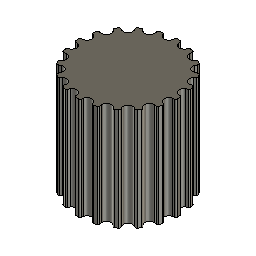
GT2-3M Generator (Autodesk Fusion 360 design; units mm, degrees)
Autodesk Fusion 360 part; units mm, degrees
sketch "Teeth" plane through (0, 0, 0) normal (0, 0, 1) x (1, 0, 0)
  circle A0 centre (0, 0) radius 9.5493
  arc A1 (0.5695, 8.5428) -> (1.2559, 7.9295) centre (1.3889, 8.769) ccw
  line L0 (0, 0) -> (0, 7.1835) construction
  line L1 (0, 0) -> (1.3889, 8.769) construction
  line L2 (0, 9.1683) -> (0, 9.5493)
  arc A2 (1.4938, 9.4317) -> (0, 9.5493) centre (0, 0) ccw
  arc A3 (0.2724, 9.1643) -> (0, 9.1683) centre (0, 0) ccw
  arc A4 (0.515, 8.919) -> (0.2724, 9.1643) centre (0.265, 8.9144) ccw
  arc A5 (0.515, 8.919) -> (0.5695, 8.5428) centre (2.0347, 8.9473) ccw
  line L3 (1.4938, 9.4317) -> (2.0963, 9.3363) construction
  line L4 (2.0347, 8.9473) -> (2.0963, 9.3363) construction
  arc A6 (1.2559, 7.9295) -> (2.0982, 8.3007) centre (1.3889, 8.769) ccw
  arc A7 (2.0982, 8.3007) -> (2.2664, 8.6416) centre (0.8297, 9.1381) ccw
  arc A8 (2.5728, 8.7999) -> (2.2664, 8.6416) centre (2.5026, 8.56) ccw
  arc A9 (2.8332, 8.7196) -> (2.5728, 8.7999) centre (0, 0) ccw
  line L5 (2.8332, 8.7196) -> (2.9509, 9.0819)
  arc A10 (2.9509, 9.0819) -> (1.4938, 9.4317) centre (0, 0) ccw
  dimension "d50" = 19.0986
  dimension "d59" = 9
  dimension "d67" = 0.381
  dimension "d68" = 0.25
  dimension "d69" = 1.521
  dimension "d71" = 0.61
  dimension "d72" = 0.85
  dimension "d73" = 1.52
  constraint coincident A0.centre L0.start
  constraint coincident A0 L2.end
  constraint parallel L0 L2
  constraint coincident A0 A2.start
  constraint collinear A1.centre A0.centre A2.start
  constraint coincident A1.centre L1.end
  constraint coincident L1 A1.end
  constraint vertical L0
  constraint coincident L0 L2.start
  constraint tangent A3 A4
  constraint tangent A4 A5
  constraint tangent A1 A5
  constraint tangent A0 L3
  constraint coincident A5.centre L4.start
  constraint coincident L3 L4.end
  constraint perpendicular L3 L4
  constraint coincident L3.end L4.end
  constraint symmetric A1 L1 A6
  constraint symmetric L1 L2.end L5.end
  constraint symmetric L1 A2.start L3.start
  constraint symmetric L1 A2 A10
  constraint symmetric L1 A1.end A6.start
  constraint symmetric L1 L2.start A9.start
  constraint symmetric L1 A3.start A8.start
  constraint symmetric L1 A3 A9
  constraint symmetric L1 A4.start A7.end
  constraint symmetric L1 A4 A8
  constraint symmetric L1 A1.start A6.end
  constraint symmetric L1 A5 A7
  measures "d50" diameter of A0
  measures "d59" angle of L0 L1
  measures "d67" distance of L2.end L2.start
  measures "d68" radius of A4
  measures "d69" distance of A2.start A1.end
  measures "d71" distance of A2.start L3.end
  measures "d72" radius of A1
  measures "d73" radius of A5
extrude "Extrude1" add sketch "Teeth" along normal mid plane 18.5
extrude "Extrude3" cut sketch "Teeth" along normal through all and the other way through all contours A0 A1 L2 A2 A3 A4 A5 A6 A7 A8 A9 L5 A10
pattern_circular "C-Pattern1" count 20 over 360 about axis through (0, 0, 0) along (0, 0, 1) of "Extrude3"
equation "p = 3 mm"
equation "Dr = 0.2 in" comment "0.13 for #25, 0.2 for #35"
equation "Ds = 1.0005 * Dr + 0.003 in"
equation "n = 20" comment "Number of Teeth"
equation "PD = n * p / 3.14159"
equation "A_angle = 35 deg + ( 60 / n ) * 1 deg"
equation "B_angle = 18 deg - ( 56 / n ) * 1 deg"
equation "ac = 0.8 * Dr"
equation "ab = 1.4 * Dr"
equation "OD = PD + 0.55 * p"
equation "d25 = width"
equation "d50 = PD"
equation "d52 = n"
equation "d59 = ( 180 / n ) * 1 deg"
equation "width = 18.5 mm"
